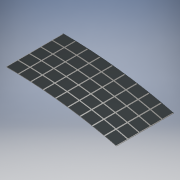
# Autodesk Inventor part: solar_panel
Saved by Autodesk Inventor 2019 (Build 230136000, 136)
## iProperties
Created: 2019-02-24
Part Number: solar_panel
Material: Steel, Carbon
Document SubType Name: Modeling
Designer: gaincarlo
Density: 7.85 g/cm^3
Appearance: Semi-Polished
Author: gaincarlo
Autodesk Inventor part; units mm, degrees
ref_plane "YZ Plane" through (0, 0, 0) normal (1, 0, 0) x (0, 1, 0)
ref_plane "XZ Plane" through (0, 0, 0) normal (0, 1, 0) x (-1, 0, 0)
ref_plane "XY Plane" through (0, 0, 0) normal (0, 0, 1) x (1, 0, 0)
sketch "Sketch1" plane through (0, 0, 0) normal (0, 0, 1) x (1, 0, 0)
  arc A0 (967.6876, 3881.1829) -> (0, 4000) centre (0, 0) ccw
  line L0 (0, 0) -> (0, 4000) construction
  line L1 (0, 0) -> (967.6876, 3881.1829) construction
  arc A1 (966.478, 3876.3314) -> (0, 3995) centre (0, 0) ccw
  line L2 (0, 4000) -> (0, 3995)
  line L3 (967.6876, 3881.1829) -> (966.478, 3876.3314)
  dimension "d2" = 8000
  dimension "d3" = 14
  dimension "d4" = 7990
  constraints: 8 end point, 4 point on circle, 2 centre point, 2 collinear, 2 point on line, 1 coincident, 1 vertical
  measures "d2" diameter of A0
  measures "d3" angle of L1 L0
  measures "d4" diameter of A1
extrude "Extrusion1" add sketch "Sketch1" along normal blind 500
ref_plane "Work Plane1" through (0, 0, 400) normal (0, 0, 1) x (1, 0, 0)
sketch "Sketch2" plane through (0, 0, 400) normal (0, 0, 1) x (1, 0, 0)
  line L0 (967.6876, 3881.1829) -> (966.478, 3876.3314) projected
  arc A0 (966.478, 3876.3314) -> (0, 3995) centre (0, 0) ccw projected
  line L1 (0, 3995) -> (0, 4000) projected
  arc A1 (967.6876, 3881.1829) -> (0, 4000) centre (0, 0) ccw projected
  arc A2 (965.7496, 3877.5435) -> (1, 3995.9999) centre (0, 0) ccw
  line L2 (965.7496, 3877.5435) -> (966.4753, 3880.4544)
  arc A3 (966.4753, 3880.4544) -> (1, 3998.9999) centre (0, 0) ccw
  line L3 (1, 3998.9999) -> (1, 3995.9999)
  dimension "d8" = 1
  constraints: 4 end point, 4 point on circle, 2 centre point, 3 other
  measures "d8" radial gap between concentric circles of A0 A2
extrude "Extrusion2" cut sketch "Sketch2" along normal mid plane 10
pattern_linear "Rectangular Pattern1" count 4 spacing 100 along (0, 0, -1) of "Extrusion2"
sketch "Sketch3" plane through (967.6876, 3881.1829, 395) normal (0.9702957, -0.2419219, 0) x (0, 0, -1)
  line L0 (300, -5) -> (300, 0) projected
  line L1 (300, 0) -> (395, 0) projected
  line L2 (395, 0) -> (395, -5) projected
  line L3 (395, -5) -> (300, -5) projected
  line L4 (200, -5) -> (200, 0) projected
  line L5 (200, 0) -> (290, 0) projected
  line L6 (290, 0) -> (290, -5) projected
  line L7 (290, -5) -> (200, -5) projected
  line L8 (100, -5) -> (100, 0) projected
  line L9 (100, 0) -> (190, 0) projected
  line L10 (190, 0) -> (190, -5) projected
  line L11 (190, -5) -> (100, -5) projected
  line L12 (90, 0) -> (90, -5) projected
  line L13 (90, -5) -> (0, -5) projected
  line L14 (0, -5) -> (0, 0) projected
  line L15 (0, 0) -> (90, 0) projected
  line L16 (-10, 0) -> (-10, -5) projected
  line L17 (-10, -5) -> (-105, -5) projected
  line L18 (-105, -5) -> (-105, 0) projected
  line L19 (-105, 0) -> (-10, 0) projected
  line L20 (-10, -4) -> (-105, -4)
  line L21 (-105, -1) -> (-10, -1)
  point P0 (395, -4000)
  dimension "d14" = 1
  constraints: 4 end point, 4 point on line
  measures "d14" distance between parallel lines of L19 L21
extrude "Extrusion3" cut sketch "Sketch3" along normal mid plane 10 contours L16 L21 L18 L19 | L16 L17 L18 L20
pattern_linear "Rectangular Pattern2" count 5 spacing 100 along (0, 0, -1) of "Extrusion3"
pattern_circular "Circular Pattern1" count 10 over 14 about axis through (0, 0, 0) along (0, 0, 1) of "Extrusion3", "Rectangular Pattern2"
equation "\"BendRadius\" = Thickness"
equation "\"BendReliefWidth\" = Thickness"
equation "\"BendReliefDepth\" = 0.5 * Thickness"
equation "\"CornerReliefSize\" = 4 * Thickness"
equation "\"MinimumRemnant\" = 2 * Thickness"
equation "\"TransitionRadius\" = BendRadius"
equation "\"JacobiRadiusSize\" = BendRadius"
equation "\"GapSize\" = Thickness"
equation "\"Thickness\" = 0.5"
body "Solid1"
